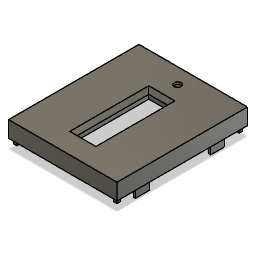
HeaterCase v8 (Autodesk Fusion 360 design; units mm, degrees)
Autodesk Fusion 360 part; units mm, degrees
sketch "Skizze8" plane through (0, 0, 0) normal (0, 1, 0) x (1, 0, 0)
  line L0 (-55.3232, 58.1924) -> (61.9768, 58.1924)
  line L1 (61.9768, 58.1924) -> (61.9768, -57.8076)
  line L2 (61.9768, -57.8076) -> (-55.3232, -57.8076)
  line L3 (-55.3232, -57.8076) -> (-55.3232, 58.1924)
  circle A0 centre (49.3768, 40.9424) radius 1.5
  circle A1 centre (-43.3232, 46.6924) radius 1.5
  circle A2 centre (-40.9232, -43.1576) radius 1.5
  circle A3 centre (47.9768, -42.4576) radius 1.5
  circle A4 centre (-43.3232, 46.6924) radius 4.3
  circle A5 centre (49.3768, 40.9424) radius 4.3
  circle A6 centre (-40.9232, -43.1576) radius 4.3
  circle A7 centre (47.9768, -42.4576) radius 4.3
  line L4 (-47.3232, 50.1924) -> (52.9268, 50.1924) construction
  line L5 (-47.3232, 50.1924) -> (-47.3232, -49.8076) construction
  line L6 (-47.3232, -49.8076) -> (53.9768, -49.8076) construction
  line L7 (53.9768, -49.8076) -> (52.9268, 50.1924) construction
  dimension "d43" = 3
  dimension "d45" = 3
  dimension "d46" = 3
  dimension "d55" = 2.8
  dimension "d56" = 2.8
  dimension "d57" = 2.8
  dimension "d58" = 2.8
  dimension "d87" = 100.25
  dimension "d88" = 100
  dimension "d89" = 101.3
  dimension "d90" = 3.5
  dimension "d91" = 4
  dimension "d92" = 6.4
  dimension "d93" = 6.65
  dimension "d94" = 7.35
  dimension "d95" = 95.3
  dimension "d96" = 96.7
  dimension "d97" = 9.25
  dimension "d98" = 8
  dimension "d99" = 8
  dimension "d100" = 8
  dimension "d101" = 8
  dimension "d102" = 3
  constraint horizontal L0
  constraint vertical L1
  constraint horizontal L2
  constraint vertical L3
  constraint perpendicular L3 L4
  constraint perpendicular L4 L5
  constraint perpendicular L5 L6
  measures "d43" diameter of A1
  measures "d45" diameter of A2
  measures "d46" diameter of A3
  measures "d87" distance of L4.start L4.end
  measures "d88" distance of L4.start L5.end
  measures "d89" distance of L5.end L6.end
  measures "d90" distance of A1.centre L4
  measures "d91" distance of A1.centre L5
  measures "d92" distance of A2.centre L5
  measures "d93" distance of A2.centre L6
  measures "d94" distance of A3.centre L6
  measures "d95" distance of A3.centre L5
  measures "d96" distance of A0.centre L5
  measures "d97" distance of A0.centre L4
  measures "d98" distance of L3 L5
  measures "d99" distance of L2 L6
  measures "d100" distance of L0 L4
  measures "d101" distance of L1 L6.end
  measures "d102" diameter of A0
extrude "Extrusion7" add sketch "Skizze8" along normal blind 9 contours A4 | A5 | A6 | A7 makes body 1 at (53.6715, 6, -40.7281) makes body 2 at (-36.6285, 6, 43.3719) makes body 3 at (-39.0285, 6, -46.4781) makes body 4 at (52.2715, 6, 42.6719)
sketch "Skizze9" plane through (0, 9, 0) normal (0, 1, 0) x (-1, 0, 0)
  circle A0 centre (40.9232, 43.1576) radius 1.5
  circle A1 centre (40.9232, 43.1576) radius 4.3
  line L0 (55.3232, 57.8076) -> (55.3232, -58.1924)
  line L1 (55.3232, -58.1924) -> (-61.9768, -58.1924)
  line L2 (-61.9768, -58.1924) -> (-61.9768, 57.8076)
  line L3 (-61.9768, 57.8076) -> (55.3232, 57.8076)
extrude "Extrusion8" add sketch "Skizze9" along normal blind 2.5 contours A0 | A1 | L0 L1 L2 L3 bodies 1 2 3 4
sketch "Skizze14" plane through (0, 11.5, 0) normal (0, 1, 0) x (-1, 0, 0)
  line L0 (-61.9768, 57.8076) -> (-61.9768, -58.1924)
  line L1 (-61.9768, -58.1924) -> (55.3232, -58.1924)
  line L2 (55.3232, -58.1924) -> (55.3232, 57.8076)
  line L3 (55.3232, 57.8076) -> (-61.9768, 57.8076)
  line L4 (47.3232, -50.1924) -> (-52.9268, -50.1924)
  line L5 (47.3232, -50.1924) -> (47.3232, 49.8076)
  line L6 (-53.9768, 49.8076) -> (-52.9268, -50.1924)
  line L7 (47.3232, 49.8076) -> (-53.9768, 49.8076)
  line L8 (7.2232, -45.6924) -> (-13.0268, -45.6924)
  line L9 (-13.0268, -45.6924) -> (-13.0268, 31.7076)
  line L10 (-13.0268, 31.7076) -> (7.2232, 31.7076)
  line L11 (7.2232, 31.7076) -> (7.2232, -45.6924)
  dimension "d103" = 40.1
  dimension "d106" = 20.25
  dimension "d107" = 4.5
  dimension "d108" = 77.4
  constraint parallel L9 L11
  constraint parallel L8 L10
  constraint parallel L5 L11
  constraint perpendicular L10 L11
  measures "d103" distance of L5 L8.start
  measures "d106" distance of L8.start L8.end
  measures "d107" distance of L4 L8
  measures "d108" distance of L8.end L9.end
extrude "Extrusion12" cut sketch "Skizze14" against normal up to surface (2.5 mm away) contours L8 L9 L10 L11 bodies 1
sketch "Skizze15" plane through (0, 9, 0) normal (0, -1, 0) x (1, 0, 0)
  line L0 (-7.2232, -45.6924) -> (-7.2232, 31.7076)
  line L1 (-7.2232, 31.7076) -> (13.0268, 31.7076)
  line L2 (13.0268, 31.7076) -> (13.0268, -45.6924)
  line L3 (13.0268, -45.6924) -> (-7.2232, -45.6924)
  circle A0 centre (-43.3232, -46.6924) radius 4.3
  circle A1 centre (49.3768, -40.9424) radius 4.3
  line L4 (61.9768, -58.1924) -> (61.9768, 57.8076)
  line L5 (61.9768, 57.8076) -> (-55.3232, 57.8076)
  line L6 (-55.3232, 57.8076) -> (-55.3232, -58.1924)
  line L7 (-55.3232, -58.1924) -> (61.9768, -58.1924)
  circle A2 centre (-40.9232, 43.1576) radius 4.3
  circle A3 centre (47.9768, 42.4576) radius 4.3
  line L8 (15.5268, -48.1924) -> (-9.7232, -48.1924)
  line L9 (-9.7232, -48.1924) -> (-9.7232, 34.2076)
  line L10 (-9.7232, 34.2076) -> (15.5268, 34.2076)
  line L11 (15.5268, 34.2076) -> (15.5268, -48.1924)
  dimension "d111" = -2.5
extrude "Extrusion13" add sketch "Skizze15" along normal blind 6 contours L8 L9 L10 L11 bodies 1
chamfer "Fase12" distance 4 angle 45 4 edges at (2.9018, 9, -48.1924) (15.5268, 9, -6.9924) (2.9018, 9, 34.2076) (-9.7232, 9, -6.9924) on bodies 1
chamfer "Fase13" distance 4 angle 45 4 edges at (-7.2232, 11.5, -6.9924) (2.9018, 11.5, -45.6924) (13.0268, 11.5, -6.9924) (2.9018, 11.5, 31.7076) on bodies 1
sketch "Skizze16" plane through (0, 11.5, 0) normal (0, 1, 0) x (-1, 0, 0)
  line L0 (-61.9768, 57.8076) -> (-61.9768, -58.1924)
  line L1 (-61.9768, -58.1924) -> (55.3232, -58.1924)
  line L2 (55.3232, -58.1924) -> (55.3232, 57.8076)
  line L3 (55.3232, 57.8076) -> (-61.9768, 57.8076)
  line L4 (11.2232, 35.7076) -> (11.2232, -49.6924)
  line L5 (11.2232, -49.6924) -> (-17.0268, -49.6924)
  line L6 (-17.0268, -49.6924) -> (-17.0268, 35.7076)
  line L7 (-17.0268, 35.7076) -> (11.2232, 35.7076)
  line L8 (55.3232, -58.1924) -> (-61.9768, -58.1924)
  line L9 (-61.9768, -58.1924) -> (-61.9768, -83.1924)
  line L10 (-61.9768, -83.1924) -> (55.3232, -83.1924)
  line L11 (55.3232, -83.1924) -> (55.3232, -58.1924)
  line L12 (-3.3268, -83.1924) -> (-3.3268, -49.6924) construction
  circle A0 centre (-3.3268, -66.4424) radius 3.75
  dimension "d116" = 25
  dimension "d117" = 7.5
  constraint perpendicular L8 L9
  constraint parallel L8 L10
  constraint parallel L9 L11
  constraint coincident L0.end L1.start
  constraint perpendicular L0 L8
  constraint coincident L1.end L2.start
  constraint midpoint L10 L12.start
  constraint coincident L5 L12.end
  constraint perpendicular L5 L12
  constraint midpoint L12 A0.centre
  measures "d116" distance of L1.end L10.end
  measures "d117" diameter of A0
extrude "Extrusion14" add sketch "Skizze16" against normal blind 2.5 contours L1 L8 L9 L10 L11 bodies 1
sketch "Skizze19" plane through (0, 9, 0) normal (0, -1, 0) x (1, 0, 0)
  circle A0 centre (3.3268, -66.4424) radius 3.75
  circle A1 centre (47.9768, 42.4576) radius 4.3
  circle A2 centre (-40.9232, 43.1576) radius 4.3
  line L0 (61.9768, -83.1924) -> (61.9768, 57.8076)
  line L1 (61.9768, 57.8076) -> (-55.3232, 57.8076)
  line L2 (-55.3232, 57.8076) -> (-55.3232, -83.1924)
  line L3 (-55.3232, -83.1924) -> (61.9768, -83.1924)
  circle A3 centre (49.3768, -40.9424) radius 4.3
  circle A4 centre (-43.3232, -46.6924) radius 4.3
  line L4 (19.5268, 38.2076) -> (19.5268, -52.1924)
  line L5 (19.5268, -52.1924) -> (-13.7232, -52.1924)
  line L6 (-13.7232, -52.1924) -> (-13.7232, 38.2076)
  line L7 (-13.7232, 38.2076) -> (19.5268, 38.2076)
  line L8 (-52.8232, -80.6924) -> (59.4768, -80.6924)
  line L9 (59.4768, -80.6924) -> (59.4768, 55.3076)
  line L10 (59.4768, 55.3076) -> (-52.8232, 55.3076)
  line L11 (-52.8232, 55.3076) -> (-52.8232, -80.6924)
  dimension "d122" = -2.5
extrude "Extrusion15" add sketch "Skizze19" along normal blind 15 contours L0 L1 L2 L3 bodies 1
sketch "Skizze20" plane through (0, -6, 0) normal (0, -1, 0) x (1, 0, 0)
  line L0 (-52.8232, -80.6924) -> (-52.8232, 55.3076)
  line L1 (-52.8232, 55.3076) -> (59.4768, 55.3076)
  line L2 (59.4768, 55.3076) -> (59.4768, -80.6924)
  line L3 (59.4768, -80.6924) -> (-52.8232, -80.6924)
  line L4 (-55.3232, -83.1924) -> (61.9768, -83.1924)
  line L5 (61.9768, -83.1924) -> (61.9768, 57.8076)
  line L6 (61.9768, 57.8076) -> (-55.3232, 57.8076)
  line L7 (-55.3232, 57.8076) -> (-55.3232, -83.1924)
  line L8 (-47.3232, 49.8076) -> (53.9768, 49.8076)
  line L9 (-47.3232, -50.1924) -> (-47.3232, 49.8076)
  line L10 (53.9768, 49.8076) -> (52.9268, -50.1924)
  line L11 (-47.3232, -50.1924) -> (52.9268, -50.1924)
  line L12 (-24.0407, -50.1924) -> (29.2037, -50.1924)
  line L13 (29.2037, -50.1924) -> (29.2037, -79.4376)
  line L14 (29.2037, -79.4376) -> (-24.0407, -79.4376)
  line L15 (-24.0407, -79.4376) -> (-24.0407, -50.1924)
  constraint perpendicular L12 L13
  constraint parallel L12 L14
  constraint parallel L13 L15
  constraint coincident L11 L12.end
  constraint parallel L11 L12
extrude "Extrusion1" add sketch "Skizze20" against normal up to surface (5.5 mm away) separate body contours L8 L9 L10 L11 L12 | L11 L12 L13 L14 L15 makes body 5 in component "PCBDummies_Display_Input"
copy_body "Körper->Berechn1" bodies 1 removing the originals makes body 6 in component "DisplayPart"
sketch "Skizze21" plane through (0, 9, 0) normal (0, -1, 0) x (1, 0, 0)
  line L0 (-52.8232, -80.6924) -> (59.4768, -80.6924)
  line L1 (59.4768, -80.6924) -> (59.4768, 55.3076)
  line L2 (59.4768, 55.3076) -> (-52.8232, 55.3076)
  line L3 (-52.8232, 55.3076) -> (-52.8232, -80.6924)
  circle A0 centre (3.3268, -66.4424) radius 3.75
  circle A1 centre (47.9768, 42.4576) radius 4.3
  circle A2 centre (-40.9232, 43.1576) radius 4.3
  circle A3 centre (49.3768, -40.9424) radius 4.3
  circle A4 centre (-43.3232, -46.6924) radius 4.3
  line L4 (19.5268, 38.2076) -> (19.5268, -52.1924)
  line L5 (19.5268, -52.1924) -> (-13.7232, -52.1924)
  line L6 (-13.7232, -52.1924) -> (-13.7232, 38.2076)
  line L7 (-13.7232, 38.2076) -> (19.5268, 38.2076)
  line L8 (59.4768, 35.3076) -> (59.4768, 20.3076)
  line L9 (59.4768, 20.3076) -> (56.4768, 20.3076)
  line L10 (56.4768, 20.3076) -> (56.4768, 35.3076)
  line L11 (56.4768, 35.3076) -> (59.4768, 35.3076)
  line L12 (59.4768, -45.6924) -> (59.4768, -60.6924)
  line L13 (59.4768, -60.6924) -> (56.4768, -60.6924)
  line L14 (56.4768, -60.6924) -> (56.4768, -45.6924)
  line L15 (56.4768, -45.6924) -> (59.4768, -45.6924)
  line L16 (3.3268, 55.3076) -> (3.3268, -105.1842) construction
  line L17 (-49.8232, 35.3076) -> (-52.8232, 35.3076)
  line L18 (-49.8232, 20.3076) -> (-49.8232, 35.3076)
  line L19 (-52.8232, 35.3076) -> (-52.8232, 20.3076)
  line L20 (-52.8232, 20.3076) -> (-49.8232, 20.3076)
  line L21 (-49.8232, -45.6924) -> (-52.8232, -45.6924)
  line L22 (-49.8232, -60.6924) -> (-49.8232, -45.6924)
  line L23 (-52.8232, -60.6924) -> (-49.8232, -60.6924)
  line L24 (59.4768, -80.6924) -> (55.4768, -80.6924)
  line L25 (55.4768, -80.6924) -> (55.4768, -76.6924)
  line L26 (55.4768, -76.6924) -> (59.4768, -76.6924)
  line L27 (59.4768, -76.6924) -> (59.4768, -80.6924)
  line L28 (59.4768, 55.3076) -> (55.4768, 55.3076)
  line L29 (55.4768, 55.3076) -> (55.4768, 51.3076)
  line L30 (55.4768, 51.3076) -> (59.4768, 51.3076)
  line L31 (59.4768, 51.3076) -> (59.4768, 55.3076)
  line L32 (-48.8232, -76.6924) -> (-52.8232, -76.6924)
  line L33 (-48.8232, -80.6924) -> (-48.8232, -76.6924)
  line L34 (-52.8232, -76.6924) -> (-52.8232, -80.6924)
  line L35 (-52.8232, -80.6924) -> (-48.8232, -80.6924)
  line L36 (-52.8232, 55.3076) -> (-48.8232, 55.3076)
  line L37 (-52.8232, 51.3076) -> (-52.8232, 55.3076)
  line L38 (-48.8232, 55.3076) -> (-48.8232, 51.3076)
  line L39 (-48.8232, 51.3076) -> (-52.8232, 51.3076)
  dimension "d127" = 3
  dimension "d128" = 15
  dimension "d129" = 20
  dimension "d130" = 15
  dimension "d131" = 3
  dimension "d132" = 20
  dimension "d135" = 4
  dimension "d136" = 4
  dimension "d137" = 4
  dimension "d138" = 4
  constraint perpendicular L8 L9
  constraint parallel L8 L10
  constraint parallel L9 L11
  constraint coincident L1 L8.end
  constraint parallel L1 L8
  constraint perpendicular L12 L13
  constraint parallel L12 L14
  constraint parallel L13 L15
  constraint coincident L1 L12.end
  constraint parallel L1 L12
  constraint midpoint L2 L16.start
  constraint perpendicular L0 L16
  constraint symmetric L8.start L16 L17.end
  constraint symmetric L8.end L16 L19.end
  constraint symmetric L9.end L16 L18.start
  constraint symmetric L10.end L16 L17.start
  constraint symmetric L12.start L16 L21.end
  constraint symmetric L12.end L16 L23.start
  constraint symmetric L13.end L16 L22.start
  constraint symmetric L14.end L16 L21.start
  constraint horizontal L24
  constraint vertical L25
  constraint horizontal L26
  constraint vertical L27
  constraint coincident L0.end L1.start
  constraint horizontal L28
  constraint vertical L29
  constraint horizontal L30
  constraint vertical L31
  constraint coincident L1.end L2.start
  constraint symmetric L16 L0.end L0.start
  constraint symmetric L16 L24.end L33.start
  constraint symmetric L16 L25.end L32.start
  constraint symmetric L16 L26.end L32.end
  constraint symmetric L16 L1.end L2.end
  constraint symmetric L16 L28.end L36.end
  constraint symmetric L16 L29.end L38.end
  constraint symmetric L16 L30.end L37.start
  measures "d127" distance of L8.start L10.end
  measures "d128" distance of L9.end L11
  measures "d129" distance of L2 L8.start
  measures "d130" distance of L12.start L12.end
  measures "d131" distance of L12.start L14.end
  measures "d132" distance of L0 L13.end
  measures "d135" distance of L0.end L24.end
  measures "d136" distance of L0.end L26.end
  measures "d137" distance of L1.end L28.end
  measures "d138" distance of L1.end L30.end
extrude "Extrusion1'" add sketch "Skizze21" along normal blind 25 contours L3 L21 L22 L23 | L3 L17 L18 L19 L20 | L1 L12 L13 L14 L15 | L1 L8 L9 L10 L11 bodies 6 in component "DisplayPart"
extrude "Extrusion2" add sketch "Skizze21" along normal blind 20 contours L0 L3 L32 L33 L34 L35 | L0 L1 L24 L25 L26 L27 | L2 L3 L36 L37 L38 L39 | L1 L2 L28 L29 L30 L31 bodies 6 in component "DisplayPart"
sketch "Skizze22" plane through (0, -6, 0) normal (0, -1, 0) x (1, 0, 0)
  line L0 (-52.8232, -80.6924) -> (-52.8232, -76.6924)
  line L1 (-52.8232, -76.6924) -> (-52.8232, -60.6924)
  line L2 (-52.8232, -60.6924) -> (-52.8232, -45.6924)
  line L3 (-52.8232, -45.6924) -> (-52.8232, 20.3076)
  line L4 (-52.8232, 20.3076) -> (-52.8232, 35.3076)
  line L5 (-52.8232, 35.3076) -> (-52.8232, 51.3076)
  line L6 (-52.8232, 51.3076) -> (-52.8232, 55.3076)
  line L7 (-52.8232, 55.3076) -> (-48.8232, 55.3076)
  line L8 (-48.8232, 55.3076) -> (55.4768, 55.3076)
  line L9 (55.4768, 55.3076) -> (59.4768, 55.3076)
  line L10 (59.4768, 55.3076) -> (59.4768, 51.3076)
  line L11 (59.4768, 51.3076) -> (59.4768, 35.3076)
  line L12 (59.4768, 35.3076) -> (59.4768, 20.3076)
  line L13 (59.4768, 20.3076) -> (59.4768, -45.6924)
  line L14 (59.4768, -45.6924) -> (59.4768, -60.6924)
  line L15 (59.4768, -60.6924) -> (59.4768, -76.6924)
  line L16 (59.4768, -76.6924) -> (59.4768, -80.6924)
  line L17 (59.4768, -80.6924) -> (55.4768, -80.6924)
  line L18 (55.4768, -80.6924) -> (-48.8232, -80.6924)
  line L19 (-48.8232, -80.6924) -> (-52.8232, -80.6924)
  line L20 (-55.3232, -83.1924) -> (61.9768, -83.1924)
  line L21 (61.9768, -83.1924) -> (61.9768, 57.8076)
  line L22 (61.9768, 57.8076) -> (-55.3232, 57.8076)
  line L23 (-55.3232, 57.8076) -> (-55.3232, -83.1924)
  line L24 (-52.8232, 51.3076) -> (-52.8232, 55.3076)
  line L25 (-52.8232, 55.3076) -> (-48.8232, 55.3076)
  line L26 (-52.8232, 35.3076) -> (-52.8232, 20.3076)
  line L27 (-52.8232, -76.6924) -> (-52.8232, -80.6924)
  line L28 (-52.8232, -80.6924) -> (-48.8232, -80.6924)
  line L29 (59.4768, -80.6924) -> (55.4768, -80.6924)
  line L30 (59.4768, -76.6924) -> (59.4768, -80.6924)
  line L31 (59.4768, -45.6924) -> (59.4768, -60.6924)
  line L32 (59.4768, 35.3076) -> (59.4768, 20.3076)
  line L33 (59.4768, 51.3076) -> (59.4768, 55.3076)
  line L34 (59.4768, 55.3076) -> (55.4768, 55.3076)
  line L35 (61.9768, 57.8076) -> (-55.3232, 57.8076)
  line L36 (-55.3232, 57.8076) -> (-55.3232, -83.1924)
  line L37 (-55.3232, -83.1924) -> (61.9768, -83.1924)
  line L38 (61.9768, -83.1924) -> (61.9768, 57.8076)
extrude "Extrusion1''" add sketch "Skizze22" along normal blind 20 separate body makes body 7 in component "MainbardAndMosfets"
sketch "Skizze23" plane through (0, 0, 35.3076) normal (0, 0, 1) x (1, 0, 0)
  line L0 (-49.8232, 9) -> (-52.8232, 9)
  line L1 (-52.8232, 9) -> (-52.8232, -6)
  line L2 (-52.8232, -6) -> (-52.8232, -16)
  line L3 (-52.8232, -16) -> (-49.8232, -16)
  line L4 (-49.8232, -16) -> (-49.8232, 9)
  line L5 (-49.8232, 9) -> (-50.8232, -16)
  dimension "d143" = 2
  constraint coincident L0.start L4.end
  constraint coincident L3 L5.end
  measures "d143" distance of L2.end L5.end
extrude "Extrusion3" cut sketch "Skizze23" against normal up to surface (96 mm away) contours L3 L4 L5 bodies 6 in component "DisplayPart"
sketch "Skizze24" plane through (0, 0, 35.3076) normal (0, 0, 1) x (1, 0, 0)
  line L0 (59.4768, 9) -> (56.4768, 9)
  line L1 (56.4768, 9) -> (56.4768, -16)
  line L2 (56.4768, -16) -> (59.4768, -16)
  line L3 (59.4768, -16) -> (59.4768, -6)
  line L4 (59.4768, -6) -> (59.4768, 9)
  line L5 (56.4768, 9) -> (57.4768, -16)
  dimension "d146" = 2
  constraint coincident L0.end L1.start
  constraint coincident L2 L5.end
  measures "d146" distance of L2.end L5.end
extrude "Extrusion4" cut sketch "Skizze24" against normal up to surface (96 mm away) contours L1 L2 L5 bodies 6 in component "DisplayPart"
component "PCBDummies_Display_Input" placed x (1, 0, 0) y (0, 1, 0) z (0, 0, 1) at (0, 0, 0)
component "DisplayPart" placed x (1, 0, 0) y (0, 1, 0) z (0, 0, 1) at (0, 0, 0)
component "MainbardAndMosfets" placed x (1, 0, 0) y (0, 1, 0) z (0, 0, 1) at (0, -0.3, 0)
equation "d103 = 40.6 mm - 0.5 mm"
